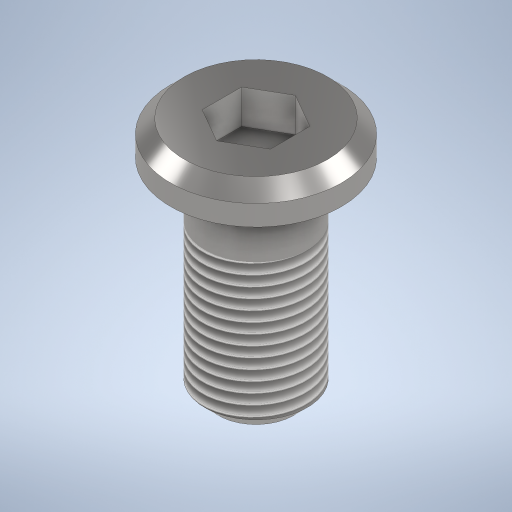
# Autodesk Inventor part: Tutorial Pt.2
Saved by Autodesk Inventor 2024.4 (Build 284460000, 460)
## iProperties
Created: 2026-06-11
Part Number: Tutorial Pt.2
Material: Stainless Steel
Document SubType Name: Modeling
Designer: stanc
Density: 8 g/cm^3
Appearance: Semi-Polished
Author: stanc
Autodesk Inventor part; units mm, degrees
ref_plane "YZ Plane" through (0, 0, 0) normal (1, 0, 0) x (0, 1, 0)
ref_plane "XZ Plane" through (0, 0, 0) normal (0, 1, 0) x (-1, 0, 0)
ref_plane "XY Plane" through (0, 0, 0) normal (0, 0, 1) x (1, 0, 0)
sketch "Sketch1" plane through (0, 0, 0) normal (0, 1, 0) x (-1, 0, 0)
  circle A0 centre (0, 0) radius 7.5
  dimension "d0" = 15
  constraints: 1 centre point, 1 coincident
  measures "d0" diameter of A0
extrude "Extrusion1" add sketch "Sketch1" along normal blind 30
chamfer "Chamfer1" distance 2 angle 45 1 edges at (7.5, 0, 0)
sketch "Sketch2" plane through (0, 30, 0) normal (0, 1, 0) x (1, 0, 0)
  circle A0 centre (0, 0) radius 12.5
  dimension "d6" = 25
  constraints: 1 centre point, 1 coincident
  measures "d6" diameter of A0
extrude "Extrusion2" add sketch "Sketch2" along normal blind 5
chamfer "Chamfer2" distance 2 angle 45 1 edges at (-12.5, 35, 0)
thread "Thread1" size "M15x1.5" class "6g" standard "ISO Metric profile" length 20
sketch "Sketch3" plane through (0, 35, 0) normal (0, 1, 0) x (1, 0, 0)
  line L0 (0, 5.7735) -> (5, 2.8868)
  line L1 (5, 2.8868) -> (5, -2.8868)
  line L2 (5, -2.8868) -> (0, -5.7735)
  line L3 (0, -5.7735) -> (-5, -2.8868)
  line L4 (-5, -2.8868) -> (-5, 2.8868)
  line L5 (-5, 2.8868) -> (0, 5.7735)
  point P0 (0, 0)
  point P1 (0, 0)
  dimension "d14" = 10
  constraints: 12 end point, 1 coincident, 13 other
  measures "d14" distance between parallel lines of L1 L4
extrude "Extrusion3" cut sketch "Sketch3" against normal blind 5
body "Solid1"
